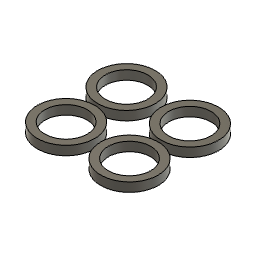
separadores v1 (Autodesk Fusion 360 design; units mm, degrees)
Autodesk Fusion 360 part; units mm, degrees
sketch "Sketch1" plane through (0, 0, 0) normal (0, 1, 0) x (1, 0, 0)
  circle A0 centre (0, 0) radius 3.5
  circle A1 centre (0, 0) radius 4.75
  dimension "d1" = 7
  dimension "d2" = 9.5
  constraint coincident A0.centre A1.centre
  measures "d1" diameter of A0
  measures "d2" diameter of A1
extrude "Extrude1" add sketch "Sketch1" along normal blind 1.5 makes body 1
copy_body "CopyPasteBodies1" bodies 1 makes body 2
move_body "Move1" bodies 2 to x (1, 0, 0) y (0, 1, 0) z (0, 0, 1) at (0, 0, 10)
copy_body "CopyPasteBodies2" bodies 2 1 makes body 3 makes body 4
move_body "Move2" bodies 3 4 to x (1, 0, 0) y (0, 1, 0) z (0, 0, 1) at (-11.5, 0, 0)
move_body "Move3" bodies 4 3 to x (1, 0, 0) y (0, 1, 0) z (0, 0, 1) at (1, 0, 0)
